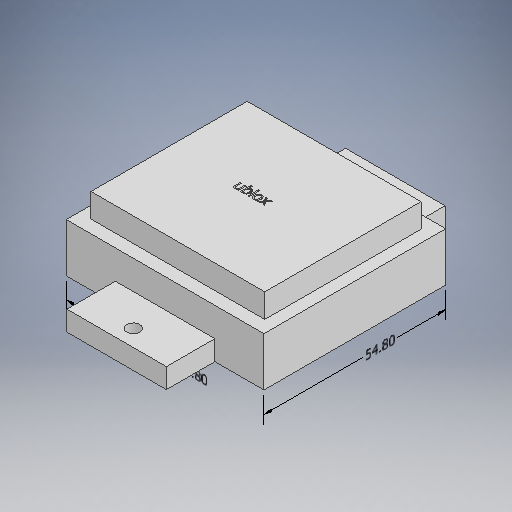
# Autodesk Inventor part: gps_antenna
Saved by Autodesk Inventor 2025.2 (Build 292293000, 293)
## iProperties
Created: 2025-03-07
Part Number: gps_antenna
Material: 일반
Document SubType Name: Modeling
Designer: jbhma
Density: 1 g/cm^3
Appearance: 기본값
Author: jbhma
Autodesk Inventor part; units mm, degrees
ref_plane "YZ Plane" through (0, 0, 0) normal (1, 0, 0) x (0, 1, 0)
ref_plane "XZ Plane" through (0, 0, 0) normal (0, 1, 0) x (-1, 0, 0)
ref_plane "XY Plane" through (0, 0, 0) normal (0, 0, 1) x (1, 0, 0)
sketch "스케치1" plane through (0, 0, 0) normal (0, 1, 0) x (-1, 0, 0)
  line L0 (0, 0) -> (-59.6, 0)
  line L1 (-59.6, 0) -> (-59.6, 54.8)
  line L2 (-59.6, 54.8) -> (0, 54.8)
  line L3 (0, 54.8) -> (0, 0)
  dimension "d0" = 59.6
  dimension "d1" = 54.8
  constraints: 8 end point, 2 parallel, 1 horizontal, 1 perpendicular
  measures "d0" distance of L1.end L2.end
  measures "d1" distance of L0.end L1.end
extrude "돌출1" add sketch "스케치1" along normal blind 14.7
sketch "스케치3" plane through (0, 14.7, 0) normal (0, 1, 0) x (1, 0, 0)
  line L0 (3.6, -3.85) -> (56, -3.85)
  line L1 (56, -3.85) -> (56, -50.95)
  line L2 (56, -50.95) -> (3.6, -50.95)
  line L3 (3.6, -50.95) -> (3.6, -3.85)
  point P0 (0, 0)
  dimension "d10" = 52.4
  dimension "d11" = 47.1
  constraints: 8 end point, 2 parallel, 1 horizontal, 1 perpendicular
  measures "d10" distance of L1.end L2.end
  measures "d11" distance of L0.end L1.end
extrude "돌출2" add sketch "스케치3" along normal blind 7.2
sketch "스케치4" plane through (0, 21.9, 0) normal (0, 1, 0) x (1, 0, 0)
  line L0 (23.4801, -25.2454) -> (33.4417, -25.2454) construction
  line L1 (33.4417, -25.2454) -> (33.4417, -28.4935) construction
  line L2 (33.4417, -28.4935) -> (23.4801, -28.4935) construction
  line L3 (23.4801, -28.4935) -> (23.4801, -25.2454) construction
  line L4 (25.5376, -28.4293) -> (25.1523, -28.4293)
  line L5 (25.1523, -28.4293) -> (25.1523, -28.1773)
  spline S0 degree 2 poles (25.1523, -28.1773) (24.9745, -28.3329) (24.6558, -28.4935) (24.4582, -28.4935) knots 0 0 0 1 2 2 2
  spline S1 degree 2 poles (24.4582, -28.4935) (24.31, -28.4935) (24.0457, -28.3947) (23.9494, -28.2885) knots 0 0 0 1 2 2 2
  spline S2 degree 2 poles (23.9494, -28.2885) (23.8506, -28.1823) (23.7419, -27.8587) (23.7419, -27.6265) knots 0 0 0 1 2 2 2
  line L6 (23.7419, -27.6265) -> (23.7419, -26.142)
  line L7 (23.7419, -26.142) -> (24.1272, -26.142)
  line L8 (24.1272, -26.142) -> (24.1272, -27.4462)
  spline S3 degree 2 poles (24.1272, -27.4462) (24.1272, -27.629) (24.1544, -27.8686) (24.2013, -27.9575) knots 0 0 0 1 2 2 2
  spline S4 degree 2 poles (24.2013, -27.9575) (24.2483, -28.0464) (24.4088, -28.1279) (24.5595, -28.1279) knots 0 0 0 1 2 2 2
  spline S5 degree 2 poles (24.5595, -28.1279) (24.7003, -28.1279) (25.0189, -27.9674) (25.1523, -27.8513) knots 0 0 0 1 2 2 2
  line L9 (25.1523, -27.8513) -> (25.1523, -26.142)
  line L10 (25.1523, -26.142) -> (25.5376, -26.142)
  line L11 (25.5376, -26.142) -> (25.5376, -28.4293)
  spline S6 degree 2 poles (28.0126, -27.2486) (28.0126, -27.8093) (27.4692, -28.4935) (27.0591, -28.4935) knots 0 0 0 1 2 2 2
  spline S7 degree 2 poles (27.0591, -28.4935) (26.8739, -28.4935) (26.6096, -28.4021) (26.4812, -28.3231) knots 0 0 0 1 2 2 2
  line L12 (26.4812, -28.3231) -> (26.4565, -28.4293)
  line L13 (26.4565, -28.4293) -> (26.0958, -28.4293)
  line L14 (26.0958, -28.4293) -> (26.0958, -25.2454)
  line L15 (26.0958, -25.2454) -> (26.4812, -25.2454)
  line L16 (26.4812, -25.2454) -> (26.4812, -26.3816)
  spline S8 degree 2 poles (26.4812, -26.3816) (26.6269, -26.2507) (26.9653, -26.0778) (27.1802, -26.0778) knots 0 0 0 1 2 2 2
  spline S9 degree 2 poles (27.1802, -26.0778) (27.568, -26.0778) (28.0126, -26.6978) (28.0126, -27.2486) knots 0 0 0 1 2 2 2
  spline S10 degree 2 poles (27.6149, -27.2782) (27.6149, -26.8682) (27.3654, -26.4434) (27.0888, -26.4434) knots 0 0 0 1 2 2 2
  spline S11 degree 2 poles (27.0888, -26.4434) (26.9332, -26.4434) (26.6121, -26.5916) (26.4812, -26.7052) knots 0 0 0 1 2 2 2
  line L17 (26.4812, -26.7052) -> (26.4812, -28.0168)
  spline S12 degree 2 poles (26.4812, -28.0168) (26.6269, -28.0884) (26.8517, -28.1477) (26.985, -28.1477) knots 0 0 0 1 2 2 2
  spline S13 degree 2 poles (26.985, -28.1477) (27.279, -28.1477) (27.6149, -27.7302) (27.6149, -27.2782) knots 0 0 0 1 2 2 2
  line L18 (28.8054, -28.4293) -> (28.4201, -28.4293)
  line L19 (28.4201, -28.4293) -> (28.4201, -25.2454)
  line L20 (28.4201, -25.2454) -> (28.8054, -25.2454)
  line L21 (28.8054, -25.2454) -> (28.8054, -28.4293)
  spline S14 degree 2 poles (31.2508, -27.2856) (31.2508, -27.8636) (30.695, -28.4935) (30.2306, -28.4935) knots 0 0 0 1 2 2 2
  spline S15 degree 2 poles (30.2306, -28.4935) (29.7539, -28.4935) (29.2081, -27.8439) (29.2081, -27.2856) knots 0 0 0 1 2 2 2
  spline S16 degree 2 poles (29.2081, -27.2856) (29.2081, -26.7126) (29.7712, -26.0778) (30.2306, -26.0778) knots 0 0 0 1 2 2 2
  spline S17 degree 2 poles (30.2306, -26.0778) (30.695, -26.0778) (31.2508, -26.7101) (31.2508, -27.2856) knots 0 0 0 1 2 2 2
  spline S18 degree 2 poles (30.8531, -27.2856) (30.8531, -26.841) (30.5295, -26.4088) (30.2306, -26.4088) knots 0 0 0 1 2 2 2
  spline S19 degree 2 poles (30.2306, -26.4088) (29.9318, -26.4088) (29.6057, -26.841) (29.6057, -27.2856) knots 0 0 0 1 2 2 2
  spline S20 degree 2 poles (29.6057, -27.2856) (29.6057, -27.7179) (29.9318, -28.1625) (30.2306, -28.1625) knots 0 0 0 1 2 2 2
  spline S21 degree 2 poles (30.2306, -28.1625) (30.5271, -28.1625) (30.8531, -27.7253) (30.8531, -27.2856) knots 0 0 0 1 2 2 2
  line L22 (33.4219, -28.4293) -> (32.9501, -28.4293)
  line L23 (32.9501, -28.4293) -> (32.3944, -27.5697)
  line L24 (32.3944, -27.5697) -> (31.8238, -28.4293)
  line L25 (31.8238, -28.4293) -> (31.3866, -28.4293)
  line L26 (31.3866, -28.4293) -> (32.1795, -27.2955)
  line L27 (32.1795, -27.2955) -> (31.394, -26.142)
  line L28 (31.394, -26.142) -> (31.8658, -26.142)
  line L29 (31.8658, -26.142) -> (32.4191, -26.9942)
  line L30 (32.4191, -26.9942) -> (32.9847, -26.142)
  line L31 (32.9847, -26.142) -> (33.4219, -26.142)
  line L32 (33.4219, -26.142) -> (32.634, -27.2708)
  line L33 (32.634, -27.2708) -> (33.4219, -28.4293)
  point P0 (0, 0)
  constraints: 2 other
extrude "돌출3" cut sketch "스케치4" against normal blind 1.55
sketch "스케치5" plane through (0, 0, 54.8) normal (0, 0, 1) x (1, 0, 0)
  line L0 (14.8, 0) -> (44.8, 0)
  line L1 (44.8, 0) -> (44.8, 6)
  line L2 (44.8, 6) -> (14.8, 6)
  line L3 (14.8, 6) -> (14.8, 0)
  point P0 (0, 0)
  dimension "d16" = 30
  dimension "d17" = 6
  constraints: 8 end point, 2 parallel, 1 horizontal, 1 perpendicular
  measures "d16" distance of L2.end L1.end
  measures "d17" distance of L1.end L0.end
sketch "스케치6" plane through (59.6, 0, 0) normal (0, 0, -1) x (-1, 0, 0)
  line L0 (44.8, 0) -> (14.8, 0)
  line L1 (14.8, 0) -> (14.8, 6)
  line L2 (14.8, 6) -> (44.8, 6)
  line L3 (44.8, 6) -> (44.8, 0)
  point P0 (59.6, 0)
  dimension "d18" = 30
  dimension "d19" = 6
  constraints: 8 end point, 2 parallel, 1 horizontal, 1 perpendicular
  measures "d18" distance of L1.end L2.end
  measures "d19" distance of L0.end L1.end
extrude "돌출4" add sketch "스케치6" along normal blind 14.6
extrude "돌출5" add sketch "스케치5" along normal blind 14.6
sketch "스케치10" plane through (14.8, 6, 54.8) normal (0, 1, 0) x (1, 0, 0)
  circle A0 centre (15, -9.6) radius 2
  point P0 (-14.8, 54.8)
  dimension "d25" = 4
  constraints: 1 centre point
  measures "d25" diameter of A0
sketch "스케치12" plane through (14.8, 6, 0) normal (0, 1, 0) x (1, 0, 0)
  circle A0 centre (15, 9.6) radius 2
  point P0 (-14.8, 0)
  dimension "d27" = 4
  constraints: 1 centre point
  measures "d27" diameter of A0
extrude "돌출6" cut sketch "스케치10" against normal blind 70.15
extrude "돌출7" cut sketch "스케치12" against normal blind 104.1
